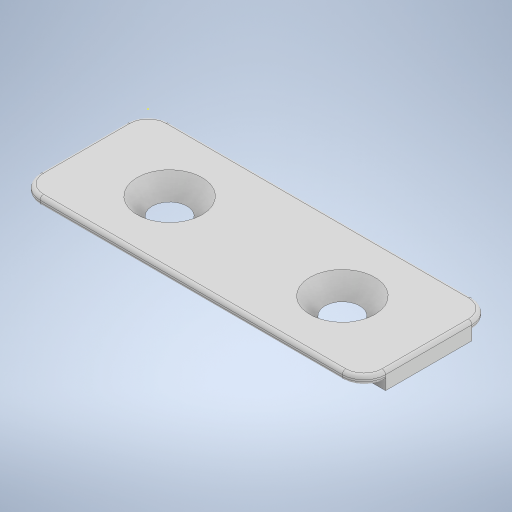
# Autodesk Inventor part: dovetail
Saved by Autodesk Inventor 2023 (Build 270158000, 158)
## iProperties
Created: 2025-10-09
Part Number: dovetail
Material: Generic
Document SubType Name: Modeling
Designer: Justin Pascual
Density: 1 g/cm^3
Appearance: Default
Author: Justin Pascual
Autodesk Inventor part; units mm, degrees
ref_plane "YZ Plane" through (0, 0, 0) normal (1, 0, 0) x (0, 1, 0)
ref_plane "XZ Plane" through (0, 0, 0) normal (0, 1, 0) x (-1, 0, 0)
sketch "Sketch1" plane through (0, 0, 0) normal (0, 1, 0) x (-1, 0, 0)
  line L0 (-3.175, 0) -> (-47.625, 0)
  line L1 (-50.8, 3.175) -> (-50.8, 15.875)
  line L2 (-47.625, 19.05) -> (-3.175, 19.05)
  line L3 (0, 15.875) -> (0, 3.175)
  arc A0 (0, 15.875) -> (-3.175, 19.05) centre (-3.175, 15.875) ccw
  arc A1 (-47.625, 19.05) -> (-50.8, 15.875) centre (-47.625, 15.875) ccw
  arc A2 (-50.8, 3.175) -> (-47.625, 0) centre (-47.625, 3.175) ccw
  arc A3 (-3.175, 0) -> (0, 3.175) centre (-3.175, 3.175) ccw
  point P0 (0, 0)
  point P1 (-50.8, 19.05)
  point P2 (-50.8, 0)
  point P3 (0, 19.05)
  dimension "d0" = 50.8
  dimension "d1" = 19.05
  dimension "d2" = 3.175
  constraints: 8 end point, 8 point on circle, 8 point on line, 8 tangent, 4 centre point, 3 equal radius, 2 parallel, 1 horizontal, 1 perpendicular
  measures "d0" distance of point (-50.8, 19.05) point (0, 19.05)
  measures "d1" distance of point (-50.8, 0) point (-50.8, 19.05)
  measures "d2" radius of A0
extrude "Extrusion1" add sketch "Sketch1" along normal blind 2.54
sketch "Sketch2" plane through (50.8, 0, 15.875) normal (1, 0, 0) x (0, 0, -1)
  line L0 (-3.175, 0) -> (-3.175, 2.54) projected
  line L1 (-3.175, 0) -> (0, 0)
  line L2 (0, 0) -> (0, 1.27)
  line L3 (0, 1.27) -> (-3.175, 1.27)
  line L4 (-3.175, 1.27) -> (-3.175, 0)
  point P0 (15.875, 0)
  dimension "d5" = 3.175
  dimension "d6" = 1.27
  constraints: 8 end point, 2 parallel, 1 horizontal, 1 perpendicular
  measures "d5" distance of L3.end L2.end
  measures "d6" distance of L2.end L1.end
extrude "Extrusion2" cut sketch "Sketch2" against normal through all
fillet "Fillet1" radius 0.508 3 edges at (25.4, 1.27, 19.05) (0.9299, 1.27, 18.1201) (49.8701, 1.27, 18.1201)
ref_plane "Work Plane1" through (3.175, 2.54, 9.525) normal (0, 0, 1) x (1, 0, 0)
mirror "Mirror1" about plane through (3.175, 2.54, 9.525) normal (0, 0, 1) of "Fillet1", "Extrusion2"
fillet "Fillet2" radius 0.508 8 edges at (0.9299, 2.54, 0.9299) (0, 2.54, 9.525) (0.9299, 2.54, 18.1201) (25.4, 2.54, 19.05) (49.8701, 2.54, 18.1201) (50.8, 2.54, 9.525) (49.8701, 2.54, 0.9299) (25.4, 2.54, 0)
sketch "Sketch3" plane through (0, 2.54, 0) normal (0, 1, 0) x (1, 0, 0)
  point P0 (0, 0)
sketch "Sketch4" plane through (0, 2.54, 0) normal (0, 1, 0) x (1, 0, 0)
  line L0 (3.175, -19.05) -> (47.625, -19.05) projected
  line L1 (0, -3.175) -> (0, -15.875) projected
  line L2 (50.8, -15.875) -> (50.8, -3.175) projected
  point P0 (0, 0)
  point P1 (12.7, -9.525)
  point P2 (38.1, -9.525)
  dimension "d11" = 9.525
  dimension "d12" = 12.7
  dimension "d13" = 12.7
  constraints: 1 horizontal alignment
  measures "d11" distance from line of L0 point (12.7, -9.525)
  measures "d12" distance from line of L1 point (12.7, -9.525)
  measures "d13" distance from line of L2 point (38.1, -9.525)
hole "Hole1" at (12.7, 2.54, 9.525) at (38.1, 2.54, 9.525) direction (0, -1, 0) diameter 2.6416 end through all countersink diameter 9.525 countersink angle 82 thread size "6-32 UNC" class "2B" standard "ANSI Unified Screw Threads"
equation "\"d13\" = d12"
body "Solid1"
